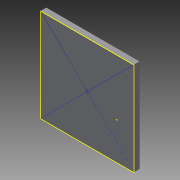
# Autodesk Inventor part: IRGlass
Saved by Autodesk Inventor 2013 (Build 170138000, 138)
## iProperties
Created: 2014-04-26
Part Number: IRGlass
Material: Generic
Document SubType Name: Modeling
Designer: spichelh
Density: 1 g/cm^3
Author: spichelh
Autodesk Inventor part; units mm, degrees
ref_plane "YZ Plane" through (0, 0, 0) normal (1, 0, 0) x (0, 1, 0)
ref_plane "XZ Plane" through (0, 0, 0) normal (0, 1, 0) x (-1, 0, 0)
ref_plane "XY Plane" through (0, 0, 0) normal (0, 0, 1) x (1, 0, 0)
sketch "Sketch1" plane through (0, 0, 0) normal (0, 0, 1) x (1, 0, 0)
  line L0 (-19.6854, 14.427) -> (4.3146, 14.427)
  line L1 (4.3146, 14.427) -> (4.3146, -9.573)
  line L2 (4.3146, -9.573) -> (-19.6854, -9.573)
  line L3 (-19.6854, -9.573) -> (-19.6854, 14.427)
  line L4 (-19.6854, 14.427) -> (4.3146, -9.573) construction
  line L5 (4.3146, 14.427) -> (-19.6854, -9.573) construction
  point P0 (0, 0)
  point P1 (-7.6854, 2.427)
  dimension "d2" = 24
  dimension "d4" = 24
  constraints: 12 end point, 2 midpoint, 2 parallel, 1 horizontal, 1 perpendicular
  measures "d2" distance of L0.start L0.end
  measures "d4" distance of L2.end L0.start
extrude "Extrusion1" add sketch "Sketch1" along normal blind 1.5
sketch "Sketch2" plane through (0, 0, 1.5) normal (0, 0, 1) x (1, 0, 0)
  line L0 (4.3146, 14.427) -> (-19.6854, 14.427) projected
  line L1 (-19.6854, 14.427) -> (-19.6854, -9.573) projected
  line L2 (-19.6854, -9.573) -> (4.3146, -9.573) projected
  line L3 (4.3146, -9.573) -> (4.3146, 14.427) projected
  line L4 (-19.6854, 14.427) -> (4.3146, -9.573) construction
  line L5 (4.3146, 14.427) -> (-19.6854, -9.573) construction
  point P0 (0, 0)
  point P1 (-7.6854, 2.427)
  constraints: 4 end point, 1 midpoint, 1 perpendicular
body "Solid1"
